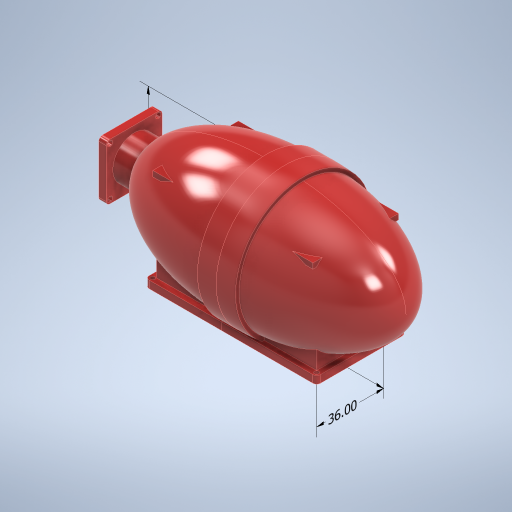
# Autodesk Inventor part: Submarino
Saved by Autodesk Inventor 2023 (Build 270158000, 158)
## iProperties
Created: 2023-03-17
Part Number: Submarino
Material: Plástico PET
Document SubType Name: Modeling
Designer: sergi
Density: 1.541 g/cm^3
Appearance: Rojo naranja
Author: sergi
Autodesk Inventor part; units mm, degrees
note: some values were not read from the file. Chosen so that the rebuilt part matches the saved one: direction of "Agujero2"; direction of "Agujero4"; direction of "Agujero5"; direction of "Agujero6"; direction of "Agujero3"; direction of "Agujero7"; direction of "Agujero8".
ref_plane "XZ Plane" through (0, 0, 0) normal (0, 1, 0) x (-1, 0, 0)
ref_plane "XY Plane" through (0, 0, 0) normal (0, 0, 1) x (1, 0, 0)
sketch "Boceto1" plane through (0, 0, 0) normal (0, 0, 1) x (1, 0, 0)
  line L0 (0, 0) -> (-65, 0)
  line L1 (0, 0) -> (0, 35)
  ellipse E0 centre (0, 0) end of major axis (-65, 0) minor radius 35
  line L2 (0, 0) -> (-62, 0)
  line L3 (0, 0) -> (0, 32)
  ellipse E1 centre (0, 0) end of major axis (-62, 0) minor radius 32
  line L4 (0, 0) -> (65, 0)
  point P0 (62, 0)
  dimension "d0" = 65
  dimension "d1" = 35
  dimension "d2" = 62
  dimension "d3" = 32
  constraints: 10 end point, 4 horizontal, 2 coincident, 2 point on line, 1 vertical, 9 other
  measures "d0" distance of L0.start L0.end
  measures "d1" distance of L0.start L1.end
  measures "d2" distance of L2.start L2.end
  measures "d3" distance of L2.start L3.end
revolve "Revolución1" add sketch "Boceto1" angle 360 about axis through (0, 0, 0) along (-1, 0, 0) contours L0 E0 L1 E1 | L1 E0 L4 E1
sketch "Boceto4" plane through (0, 0, 0) normal (0, 1, 0) x (-1, 0, 0)
  line L0 (-35, -18) -> (35, -18)
  line L1 (35, -18) -> (35, 18)
  line L2 (35, 18) -> (-35, 18)
  line L3 (-35, 18) -> (-35, -18)
  line L4 (-35, -18) -> (35, 18) construction
  line L5 (35, -18) -> (-35, 18) construction
  line L6 (-19.5, -14.5) -> (19.5, 14.5) construction
  line L7 (19.5, -14.5) -> (-19.5, 14.5) construction
  line L8 (-38, -21) -> (38, -21)
  line L9 (38, -21) -> (38, 21)
  line L10 (38, 21) -> (-38, 21)
  line L11 (-38, 21) -> (-38, -21)
  line L12 (-38, -21) -> (38, 21) construction
  line L13 (38, -21) -> (-38, 21) construction
  point P0 (0, 0)
  dimension "d21" = 76
  dimension "d22" = 42
  dimension "d44" = 3
  dimension "d45" = 3
  constraints: 28 end point, 6 midpoint, 4 parallel, 2 horizontal, 2 perpendicular
  measures "d21" distance of L10.end L9.end
  measures "d22" distance of L10.end L8.start
  measures "d44" distance between parallel lines of L10 L2
  measures "d45" distance between parallel lines of L9 L1
extrude "Extrusión1" add sketch "Boceto4" along normal blind 22 and the other way blind 33
extrude "Extrusión2" cut sketch "Boceto4" along normal blind 15 and the other way blind 35 contours L3 L2 L1 L0
sketch "Boceto6" plane through (0, 0, 0) normal (0, 0, 1) x (1, 0, 0)
  point P0 (0, 0)
ref_plane "Plano de trabajo1" through (-60, 0, 0) normal (1, 0, 0) x (0, 1, 0)
sketch "Boceto9" plane through (-60, 0, 0) normal (1, 0, 0) x (0, 1, 0)
  circle A0 centre (0, 0) radius 11.5
  circle A1 centre (0, 0) radius 8.5
  dimension "d46" = 23
  dimension "d49" = 3
  constraints: 2 centre point, 2 coincident
  measures "d46" diameter of A0
  measures "d49" radial gap between concentric circles of A0 A1
extrude "Extrusión5" cut sketch "Boceto9" against normal blind 30 contours A0 | A1
extrude "Extrusión7" cut sketch "Boceto9" along normal blind 10 contours A1
extrude "Extrusión8" add sketch "Boceto9" along normal mid plane 30
sketch "Boceto10" plane through (-75, 0, 0) normal (-1, 0, 0) x (0, 0, 1)
  line L0 (13, -15) -> (-13, -15)
  line L1 (-15, -13) -> (-15, 13)
  line L2 (-13, 15) -> (13, 15)
  line L3 (15, 13) -> (15, -13)
  line L4 (0, 32) -> (0, 0) projected
  line L5 (15, -15) -> (-15, 15) construction
  line L6 (-15, -15) -> (15, 15) construction
  circle A0 centre (0, 0) radius 11.5
  arc A1 (-13, 15) -> (-15, 13) centre (-13, 13) ccw
  arc A2 (-15, -13) -> (-13, -15) centre (-13, -13) ccw
  arc A3 (13, -15) -> (15, -13) centre (13, -13) ccw
  arc A4 (15, 13) -> (13, 15) centre (13, 13) ccw
  point P0 (0, 11.5)
  dimension "d56" = 30
  dimension "d57" = 30
  dimension "d104" = 2
  constraints: 12 end point, 8 point on circle, 8 point on line, 8 tangent, 5 centre point, 3 equal radius, 2 midpoint, 2 parallel, 1 coincident, 1 horizontal, 1 perpendicular
  measures "d56" distance of L5.end L6.end
  measures "d57" distance of L6.start L5.end
  measures "d104" radius of A1
extrude "Extrusión9" add sketch "Boceto10" against normal blind 4
sketch "Boceto12" plane through (0, 22, 0) normal (0, 1, 0) x (1, 0, 0)
  line L0 (-38, 21) -> (38, -21) construction
  line L1 (35, 20) -> (-35, -20) construction
  line L2 (-38, -23) -> (38, -23)
  line L3 (38, -23) -> (38, 23)
  line L4 (38, 23) -> (-38, 23)
  line L5 (-38, 23) -> (-38, -23)
  line L6 (-38, -23) -> (38, 23) construction
  line L7 (38, -23) -> (-38, 23) construction
  point P0 (0, 0)
  dimension "d80" = 76
  dimension "d81" = 46
  constraints: 16 end point, 4 midpoint, 2 parallel, 1 horizontal, 1 perpendicular
  measures "d80" distance of L3.end L4.end
  measures "d81" distance of L4.end L2.start
extrude "Extrusión10" add sketch "Boceto12" against normal blind 3
sketch "Boceto14" plane through (0, -33, 0) normal (0, -1, 0) x (1, 0, 0)
  line L0 (38, 21) -> (-38, 21) projected
  line L1 (38, -21) -> (-38, -21)
  line L2 (-38, -21) -> (-38, 21)
  line L3 (-38, 21) -> (38, 21)
  line L4 (38, 21) -> (38, -21)
  line L5 (38, -21) -> (-38, 21) construction
  line L6 (-38, -21) -> (38, 21) construction
  line L7 (39, -24) -> (-39, -24)
  line L8 (-41, -22) -> (-41, 22)
  line L9 (-39, 24) -> (39, 24)
  line L10 (41, 22) -> (41, -22)
  line L11 (41, -24) -> (-41, 24) construction
  line L12 (-41, -24) -> (41, 24) construction
  arc A0 (-39, 24) -> (-41, 22) centre (-39, 22) ccw
  arc A1 (41, 22) -> (39, 24) centre (39, 22) ccw
  arc A2 (39, -24) -> (41, -22) centre (39, -22) ccw
  arc A3 (-41, -22) -> (-39, -24) centre (-39, -22) ccw
  point P0 (0, 0)
  dimension "d82" = 3
  dimension "d83" = 3
  dimension "d99" = 2
  dimension "d140" = 82
  dimension "d141" = 48
  constraints: 24 end point, 8 point on circle, 8 point on line, 8 tangent, 4 centre point, 4 midpoint, 4 parallel, 3 equal radius, 2 horizontal, 2 perpendicular
  measures "d82" distance between parallel lines of L7 L1
  measures "d83" distance between parallel lines of L10 L4
  measures "d99" radius of A0
  measures "d140" distance between parallel lines of L8 L10
  measures "d141" distance between parallel lines of L9 L7
extrude "Extrusión11" add sketch "Boceto14" against normal blind 4
sketch "Boceto16" plane through (0, -33, 0) normal (0, -1, 0) x (1, 0, 0)
  line L0 (-35, 18) -> (35, 18) projected
  line L1 (35, -18) -> (-35, -18)
  line L2 (-35, -18) -> (-35, 18)
  line L3 (-35, 18) -> (35, 18)
  line L4 (35, 18) -> (35, -18)
  line L5 (35, -18) -> (-35, 18) construction
  line L6 (-35, -18) -> (35, 18) construction
  line L7 (-38, -21) -> (38, -21)
  line L8 (38, -21) -> (38, 21)
  line L9 (38, 21) -> (-38, 21)
  line L10 (-38, 21) -> (-38, -21)
  line L11 (-38, -21) -> (38, 21) construction
  line L12 (38, -21) -> (-38, 21) construction
  point P0 (0, 0)
  dimension "d100" = 3
  dimension "d101" = 3
  constraints: 24 end point, 4 midpoint, 4 parallel, 2 horizontal, 2 perpendicular
  measures "d100" distance between parallel lines of L8 L4
  measures "d101" distance between parallel lines of L9 L0
extrude "Extrusión13" cut sketch "Boceto16" against normal blind 1
sketch "Boceto17" plane through (-75, 0, 0) normal (-1, 0, 0) x (0, 0, 1)
  line L0 (10, -10) -> (-10, -10)
  line L1 (-10, -10) -> (-10, 10)
  line L2 (-10, 10) -> (10, 10)
  line L3 (10, 10) -> (10, -10)
  line L4 (0, 32) -> (0, 0) projected
  line L5 (10, -10) -> (-10, 10) construction
  line L6 (-10, -10) -> (10, 10) construction
  line L7 (11, -11) -> (-11, -11)
  line L8 (-11, -11) -> (-11, 11)
  line L9 (-11, 11) -> (11, 11)
  line L10 (11, 11) -> (11, -11)
  line L11 (11, -11) -> (-11, 11) construction
  line L12 (-11, -11) -> (11, 11) construction
  point P0 (0, 11.5)
  dimension "d105" = 1
  dimension "d106" = 1
  dimension "d107" = 10
  constraints: 24 end point, 4 midpoint, 4 parallel, 2 horizontal, 2 perpendicular, 1 point on line
  measures "d105" distance between parallel lines of L9 L2
  measures "d106" distance between parallel lines of L10 L3
  measures "d107" distance from line of L4.end L3
extrude "Extrusión14" cut sketch "Boceto17" against normal blind 1
sketch "Boceto19" plane through (-71, 0, 0) normal (1, 0, 0) x (0, 0, -1)
  point P0 (13, -13)
  point P1 (13, 13)
hole "Agujero2" at (-71, -13, -13) at (-71, 13, -13) direction (-1, 0, 0) diameter 2.9 depth 4
sketch "Boceto21" plane through (-71, 0, 0) normal (1, 0, 0) x (0, 0, -1)
  point P0 (-13, -13)
hole "Agujero4" at (-71, -13, 13) direction (-1, 0, 0) diameter 2.9 depth 4
sketch "Boceto22" plane through (0, -29, 0) normal (0, 1, 0) x (1, 0, 0)
  point P0 (39, 22)
hole "Agujero5" at (39, -29, -22) direction (0, -1, 0) diameter 2.4 depth 4
sketch "Boceto23" plane through (0, -29, 0) normal (0, 1, 0) x (1, 0, 0)
  point P0 (39, -22)
hole "Agujero6" at (39, -29, 22) direction (0, -1, 0) diameter 2.4 depth 4
sketch "Boceto20" plane through (-71, 0, 0) normal (1, 0, 0) x (0, 0, -1)
  point P0 (-13, 13)
hole "Agujero3" at (-71, 13, 13) direction (-1, 0, 0) diameter 2.9 depth 4
sketch "Boceto24" plane through (0, -29, 0) normal (0, 1, 0) x (1, 0, 0)
  point P0 (-39, 22)
hole "Agujero7" at (-39, -29, -22) direction (0, -1, 0) diameter 2.4 depth 4
sketch "Boceto25" plane through (0, -29, 0) normal (0, 1, 0) x (1, 0, 0)
  point P0 (-39, -22)
hole "Agujero8" at (-39, -29, 22) direction (0, -1, 0) diameter 2.4 depth 4
sketch "Boceto13" plane through (0, 0, 0) normal (0, 0, 1) x (1, 0, 0)
  point P0 (0, 0)
sketch "Boceto26" plane through (0, 0, 0) normal (1, 0, 0) x (0, 1, 0)
  point P0 (0, 0)
sketch "Boceto29" plane through (0, 0, 0) normal (1, 0, 0) x (0, 1, 0)
  point P0 (0, 0)
split body "Dividir1" result two bodies by plane through (0, 0, 0) normal (1, 0, 0) first body at (6.8605, 29.4409, -17.6061)
move or copy body "Desplazar1" bodies to move or copy 2 copy no translate (10, 0, 0)
sketch "Boceto30" plane through (10, -32, -18) normal (-1, 0, 0) x (0, 0, 1)
  line L0 (18, 32) -> (18, 67) projected
  arc A0 (36, 1.9833) -> (0, 1.9833) centre (18, 32) ccw
  line L1 (36, 0) -> (36, 51) projected
  line L2 (0, 51) -> (0, 0) projected
  arc A1 (36, -0.3265) -> (0, -0.3265) centre (18, 32) ccw
  line L3 (0, 1.9833) -> (0, -0.3265)
  line L4 (36, -0.3265) -> (36, 1.9833)
  dimension "d176" = 70
  dimension "d177" = 74
  constraints: 4 end point, 4 point on circle, 4 point on line, 2 centre point, 2 coincident, 1 collinear, 1 vertical
  measures "d176" diameter of A0
  measures "d177" diameter of A1
extrude "Extrusión16" add sketch "Boceto30" along normal blind 10 bodies 2
sketch "Boceto31" plane through (10, -32, -18) normal (1, 0, 0) x (0, 0, -1)
  arc A0 (0, 1.9833) -> (-36, 1.9833) centre (-18, 32) ccw projected
  arc A1 (0, 1.9833) -> (-36, 1.9833) centre (-18, 32) ccw
  line L0 (-18, 32) -> (-18, 64) projected
  arc A2 (0, -0.3265) -> (-36, -0.3265) centre (-18, 32) ccw
  line L1 (-36, -0.3265) -> (-36, 1.9833)
  line L2 (0, -0.3265) -> (0, 1.9833) projected
  line L3 (0, 1.9833) -> (0, -0.3265)
  constraints: 4 end point, 4 point on circle, 2 centre point, 2 coincident, 1 vertical
sketch "Boceto32" plane through (0, 0, 0) normal (0, 0, 1) x (1, 0, 0)
  ellipse E0 centre (10, 0) end of major axis (-55, 0) minor radius 35 (75, 0) -> (10, 35) ccw projected
  line L0 (0, 0) -> (0, 35.3464)
  line L1 (0, 37) -> (0, -32.3265) projected
  line L2 (0, 0) -> (0, 37)
  line L3 (0, 0) -> (75, 0)
  line L4 (0, -30.0167) -> (0, 35) projected
  line L5 (10, 37) -> (0, 37) projected
  line L6 (0, 0) -> (75, 0)
  line L7 (10, 0) -> (10, 35)
  ellipse E1 centre (10, 0) end of major axis (75, 0) minor radius 35
  line L8 (10, 0) -> (10, 37)
  line L9 (10, 37) -> (10, -29) projected
  ellipse E2 centre (10, 0) end of major axis (75, 0) minor radius 37
  line L10 (10, -24.1454) -> (10, 19) projected
  line L11 (10, 35) -> (10, 37)
  line L12 (19.9696, 36.5622) -> (19.9696, 34.5859)
  point P0 (10, 35)
  dimension "d182" = 75
  dimension "d183" = 35
  dimension "d184" = 37
  constraints: 16 end point, 4 coincident, 4 vertical, 3 perpendicular, 2 horizontal, 1 point on line, 11 other
  measures "d182" distance of L0.start L3.end
  measures "d183" distance of L7.start L7.end
  measures "d184" distance of L8.start L5.start
revolve "Revolución4" add sketch "Boceto32" angle 295 mid plane about axis through (0, 0, 0) along (1, 0, 0) bodies 2 contours E0 L8 E2 L12
thread "Rosca1" size "G 1-11" standard "BSP Pipe Threads" length 7.4
sketch "Boceto33" plane through (0, -32, 18) normal (1, 0, 0) x (0, 0, -1)
  circle A0 centre (18, 32) radius 32
  circle A1 centre (18, 32) radius 35
  line L0 (-3, 3) -> (-3, 4) projected
  line L1 (-3, 4) -> (-3, 7.8546)
  line L2 (39, 12.8865) -> (39, 3) projected
  line L3 (39, 4) -> (39, 7.9433)
  point P0 (39, 7.8546)
  dimension "d188" = 64
  dimension "d189" = 70
  constraints: 4 end point, 2 coincident, 1 centre point, 1 collinear, 1 midpoint, 1 point on circle, 1 point on line, 3 other
  measures "d189" diameter of A1
extrude "Extrusión17" add sketch "Boceto33" along normal blind 10 contours A0 L1 A1 L2 picked at (-11.1465, 16.8825) bodies 3
thread "Rosca2" size "G 1-11" class "A" standard "BSP Pipe Threads" length 7.4
sketch "Boceto36" plane through (0, -32, 18) normal (1, 0, 0) x (0, 0, -1)
  line L0 (-3, 51) -> (-3, 54)
  line L1 (0.0466, 54) -> (-5, 54) projected
  line L2 (-3, 3) -> (-3, 12.8865) projected
  line L3 (-3, 51) -> (-3, 3)
  line L4 (-3, 3) -> (-6, 3)
  line L5 (-3, -1) -> (-6, -1) projected
  line L6 (-6, 3) -> (-6, -1)
  line L7 (42, -1) -> (39, -1) projected
  line L8 (42, -1) -> (42, 3)
  line L9 (42, 3) -> (39, 3)
  line L10 (39, 51) -> (39, 7.8546) projected
  line L11 (39, 3) -> (39, 51)
  line L12 (41, 54) -> (41, 51) projected
  line L13 (39, 51) -> (39, 54)
  line L14 (41, 54) -> (35.9534, 54) projected
  line L15 (-3, 54) -> (39, 54)
  line L16 (0, 0) -> (0, 51) projected
  line L17 (0, 51) -> (35.9534, 51)
  line L18 (39, -1) -> (39, 0) projected
  line L19 (36, 0) -> (39, 0)
  line L20 (39, 0) -> (39, -1)
  line L21 (-3, -1) -> (-3, 0) projected
  line L22 (-3, -1) -> (-3, 0)
  line L23 (-3, 0) -> (0, 0)
  line L24 (39, 0) -> (-3, 0) projected
  line L25 (0, 51) -> (0, 0)
  line L26 (-6, -1) -> (-3, -1)
  line L27 (39, -1) -> (42, -1)
  line L28 (42, 3) -> (42, -1)
  line L29 (39, 0) -> (36, 0) projected
  line L30 (36, 0) -> (36, 51)
  line L31 (18, 43.5) -> (18, 64) projected
  line L32 (18, 51) -> (18, 53.75)
  arc A0 (39, 4) -> (-3, 4) centre (18, 32) ccw projected
  line L33 (-3, 4) -> (0, 4)
  line L34 (0, 51) -> (0, 0) projected
  point P0 (18, 54)
  constraints: 42 end point, 7 point on line, 6 collinear, 4 perpendicular, 4 vertical, 3 horizontal, 1 midpoint
extrude "Extrusión18" add sketch "Boceto36" along normal blind 10 contours L0 L1 L15 L31 L17 L16 L33 L2 L3 bodies 3
sketch "Boceto37" plane through (0, -32, -18) normal (1, 0, 0) x (0, 0, -1)
  line L0 (-18, 54) -> (5, 54) projected
  line L1 (-18, 54) -> (-18, 51) projected
  line L2 (-18, 54) -> (-18, 51)
  line L3 (0, 51) -> (-36, 51) projected
  line L4 (-18, 51) -> (0, 51)
  line L5 (0, 0) -> (0, 51) projected
  line L6 (0, 51) -> (0, 0)
  line L7 (3, 0) -> (0, 0) projected
  line L8 (0, 0) -> (3, 0)
  line L9 (3, 0) -> (3, -1)
  line L10 (3, -1) -> (6, -1)
  line L11 (6, -1) -> (6, 3) projected
  line L12 (6, -1) -> (6, 3)
  line L13 (6, 3) -> (3, 3)
  line L14 (3, 51) -> (3, 7.8546) projected
  line L15 (3, 3) -> (3, 51)
  line L16 (5, 51) -> (3, 51) projected
  line L17 (3, 51) -> (5, 51)
  line L18 (5, 51) -> (5, 54)
  line L19 (5, 54) -> (-18, 54)
  arc A0 (3, 4) -> (-39, 4) centre (-18, 32) ccw projected
  line L20 (3, 4) -> (0, 4)
  point P0 (3, 7.8546)
  constraints: 26 end point, 11 perpendicular, 1 collinear, 1 point on line, 1 vertical
extrude "Extrusión19" add sketch "Boceto37" along normal blind 10 contours L0 L18 L16 L14 L15 L20 L5 L3 L1 bodies 3
sketch "Boceto38" plane through (10, -33, -24) normal (-1, 0, 0) x (0, 0, 1)
  line L0 (0, 0) -> (0, 4) projected
  line L1 (3, 0) -> (3, 1) projected
  line L2 (0, 0) -> (3, 0)
  line L3 (3, 0) -> (3, 1)
  line L4 (3, 1) -> (5.4258, 1)
  arc A0 (42, 0.6735) -> (6, 0.6735) centre (24, 33) ccw projected
  line L5 (2, 4) -> (0, 4) projected
  line L6 (0, 0) -> (0, 4)
  arc A1 (46.9783, 4) -> (1.0217, 4) centre (24, 33) ccw projected
  line L7 (0, 4) -> (1.0217, 4)
  arc A2 (1.0217, 4) -> (5.4258, 1) centre (24, 33) ccw
  arc A3 (42, 0.6735) -> (42.5742, 1) centre (24, 33) ccw projected
  line L8 (45, 1) -> (45, 0) projected
  line L9 (42.5742, 1) -> (45, 1)
  line L10 (45, 1) -> (45, 0)
  line L11 (46, 0) -> (48, 0) projected
  line L12 (45, 0) -> (48, 0)
  line L13 (48, 4) -> (46, 4) projected
  line L14 (48, 0) -> (48, 4)
  line L15 (48, 4) -> (46, 4)
  point P0 (24, 33)
  point P1 (1.0217, 4)
  constraints: 20 end point, 7 perpendicular, 3 point on circle, 2 horizontal, 1 centre point, 1 concentric
extrude "Extrusión20" add sketch "Boceto38" along normal blind 10 bodies 2
